Autodesk Inventor part; units mm, degrees
(part 2 of 5)
sketch "スケッチ2" plane through (0, 0, 0) normal (0, 0, 1) x (1, 0, 0)
  arc A0 (152.8433, 93.1355) -> (152.2497, 92.5446) centre (153.1871, 92.1964) ccw
  arc A1 (144.7503, 92.5446) -> (152.2497, 92.5446) centre (148.5, 93.9374) ccw
  arc A2 (144.7503, 92.5446) -> (144.1567, 93.1355) centre (143.8129, 92.1964) ccw
  arc A3 (143.2473, 93.5091) -> (144.1567, 93.1355) centre (148.5, 105) ccw
  arc A4 (142.7704, 93.9677) -> (143.2473, 93.5091) centre (143.663, 94.4186) ccw
  arc A5 (141.9213, 97.4341) -> (142.7704, 93.9677) centre (149.832, 97.5348) ccw
  arc A6 (141.9213, 97.4341) -> (140.9341, 98.4213) centre (140.9213, 97.4213) ccw
  arc A7 (137.4677, 99.2704) -> (140.9341, 98.4213) centre (141.0348, 106.332) ccw
  arc A8 (137.0091, 99.7473) -> (137.4677, 99.2704) centre (137.9186, 100.163) ccw
  arc A9 (136.6355, 100.6567) -> (137.0091, 99.7473) centre (148.5, 105) ccw
  arc A10 (136.6355, 100.6567) -> (136.0446, 101.2503) centre (135.6964, 100.3129) ccw
  arc A11 (136.0446, 108.7497) -> (136.0446, 101.2503) centre (137.4374, 105) ccw
  arc A12 (136.0446, 108.7497) -> (136.6355, 109.3433) centre (135.6964, 109.6871) ccw
  arc A13 (137.0091, 110.2527) -> (136.6355, 109.3433) centre (148.5, 105) ccw
  arc A14 (137.4677, 110.7296) -> (137.0091, 110.2527) centre (137.9186, 109.837) ccw
  arc A15 (140.9341, 111.5787) -> (137.4677, 110.7296) centre (141.0348, 103.668) ccw
  arc A16 (140.9341, 111.5787) -> (141.9213, 112.5659) centre (140.9213, 112.5787) ccw
  arc A17 (142.7704, 116.0323) -> (141.9213, 112.5659) centre (149.832, 112.4652) ccw
  arc A18 (143.2473, 116.4909) -> (142.7704, 116.0323) centre (143.663, 115.5814) ccw
  arc A19 (144.1567, 116.8645) -> (143.2473, 116.4909) centre (148.5, 105) ccw
  arc A20 (144.1567, 116.8645) -> (144.7503, 117.4554) centre (143.8129, 117.8036) ccw
  arc A21 (152.2497, 117.4554) -> (144.7503, 117.4554) centre (148.5, 116.0626) ccw
  arc A22 (152.2497, 117.4554) -> (152.8433, 116.8645) centre (153.1871, 117.8036) ccw
  arc A23 (153.7527, 116.4909) -> (152.8433, 116.8645) centre (148.5, 105) ccw
  arc A24 (154.2296, 116.0323) -> (153.7527, 116.4909) centre (153.337, 115.5814) ccw
  arc A25 (155.0787, 112.5659) -> (154.2296, 116.0323) centre (147.168, 112.4652) ccw
  arc A26 (155.0787, 112.5659) -> (156.0659, 111.5787) centre (156.0787, 112.5787) ccw
  arc A27 (159.5323, 110.7296) -> (156.0659, 111.5787) centre (155.9652, 103.668) ccw
  arc A28 (159.9909, 110.2527) -> (159.5323, 110.7296) centre (159.0814, 109.837) ccw
  arc A29 (160.3645, 109.3433) -> (159.9909, 110.2527) centre (148.5, 105) ccw
  arc A30 (160.3645, 109.3433) -> (160.9554, 108.7497) centre (161.3036, 109.6871) ccw
  arc A31 (160.9554, 101.2503) -> (160.9554, 108.7497) centre (159.5626, 105) ccw
  arc A32 (160.9554, 101.2503) -> (160.3645, 100.6567) centre (161.3036, 100.3129) ccw
  arc A33 (159.9909, 99.7473) -> (160.3645, 100.6567) centre (148.5, 105) ccw
  arc A34 (159.5323, 99.2704) -> (159.9909, 99.7473) centre (159.0814, 100.163) ccw
  arc A35 (156.0659, 98.4213) -> (159.5323, 99.2704) centre (155.9652, 106.332) ccw
  arc A36 (156.0659, 98.4213) -> (155.0787, 97.4341) centre (156.0787, 97.4213) ccw
  arc A37 (154.2296, 93.9677) -> (155.0787, 97.4341) centre (147.168, 97.5348) ccw
  arc A38 (153.7527, 93.5091) -> (154.2296, 93.9677) centre (153.337, 94.4186) ccw
  arc A39 (152.8433, 93.1355) -> (153.7527, 93.5091) centre (148.5, 105) ccw
  circle A40 centre (148.5, 105) radius 3
  circle A41 centre (148.5, 116.0626) radius 1.25
  circle A42 centre (137.4374, 105) radius 1.25
  circle A43 centre (159.5626, 105) radius 1.25
  circle A44 centre (148.5, 93.9374) radius 1.25
  arc A45 (148.106, 135.7475) -> (147.9566, 136.3017) centre (140.7163, 134.0527) ccw projected
  arc A46 (148.894, 135.7475) -> (148.106, 135.7475) centre (148.5, 105) ccw projected
  arc A47 (149.0434, 136.3017) -> (148.894, 135.7475) centre (156.2837, 134.0527) ccw projected
  arc A48 (149.3046, 137.0392) -> (149.0434, 136.3017) centre (158.5049, 133.3653) ccw projected
  arc A49 (149.7251, 137.9773) -> (149.3046, 137.0392) centre (160.7701, 132.4624) ccw projected
  arc A50 (150.5131, 137.9385) -> (149.7251, 137.9773) centre (148.5, 105) ccw projected
  arc A51 (150.8397, 136.9638) -> (150.5131, 137.9385) centre (138.9807, 133.5328) ccw projected
  arc A52 (151.0273, 136.2043) -> (150.8397, 136.9638) centre (141.3236, 134.2093) ccw projected
  arc A53 (151.1217, 135.638) -> (151.0273, 136.2043) centre (143.6015, 134.6758) ccw projected
  arc A54 (151.9058, 135.5608) -> (151.1217, 135.638) centre (148.5, 105) ccw projected
  arc A55 (152.1089, 136.0978) -> (151.9058, 135.5608) centre (159.0939, 133.1499) ccw projected
  arc A56 (152.4411, 136.8061) -> (152.1089, 136.0978) centre (161.237, 132.248) ccw projected
  arc A57 (152.9516, 137.6984) -> (152.4411, 136.8061) centre (163.4028, 131.1274) ccw projected
  arc A58 (153.7319, 137.5826) -> (152.9516, 137.6984) centre (148.5, 105) ccw projected
  arc A59 (153.9614, 136.5805) -> (153.7319, 137.5826) centre (141.8233, 134.3285) ccw projected
  arc A60 (154.0737, 135.8063) -> (153.9614, 136.5805) centre (144.2211, 134.7721) ccw projected
  arc A61 (154.1121, 135.2335) -> (154.0737, 135.8063) centre (146.5338, 135.013) ccw projected
  arc A62 (154.8849, 135.0798) -> (154.1121, 135.2335) centre (148.5, 105) ccw projected
  arc A63 (155.1396, 135.5943) -> (154.8849, 135.0798) centre (161.802, 131.976) ccw projected
  arc A64 (155.5397, 136.2666) -> (155.1396, 135.5943) centre (163.8464, 130.8684) ccw projected
  arc A65 (156.1351, 137.1046) -> (155.5397, 136.2666) centre (165.892, 129.5409) ccw projected
  arc A66 (156.9004, 136.9129) -> (156.1351, 137.1046) centre (148.5, 105) ccw projected
  arc A67 (157.0305, 135.8932) -> (156.9004, 136.9129) centre (144.7301, 134.8417) ccw projected
  arc A68 (157.0664, 135.1116) -> (157.0305, 135.8932) centre (147.1599, 135.0481) ccw projected
  arc A69 (157.0485, 134.5379) -> (157.0664, 135.1116) centre (149.485, 135.0612) ccw projected
  arc A70 (157.8025, 134.3091) -> (157.0485, 134.5379) centre (148.5, 105) ccw projected
  arc A71 (158.1064, 134.7962) -> (157.8025, 134.3091) centre (164.3821, 130.5422) ccw projected
  arc A72 (158.5704, 135.426) -> (158.1064, 134.7962) centre (166.3081, 129.2396) ccw projected
  arc A73 (159.2452, 136.2016) -> (158.5704, 135.426) centre (168.2137, 127.718) ccw projected
  arc A74 (159.988, 135.9358) -> (159.2452, 136.2016) centre (148.5, 105) ccw projected
  arc A75 (160.0175, 134.9083) -> (159.988, 135.9358) centre (147.6733, 135.0675) ccw projected
  arc A76 (159.9766, 134.127) -> (160.0175, 134.9083) centre (150.1116, 135.0348) ccw projected
  arc A77 (159.9026, 133.5577) -> (159.9766, 134.127) centre (152.4268, 134.8199) ccw projected
  arc A78 (160.6305, 133.2562) -> (159.9026, 133.5577) centre (148.5, 105) ccw projected
  arc A79 (160.9807, 133.7111) -> (160.6305, 133.2562) centre (166.8092, 128.8625) ccw projected
  arc A80 (161.5042, 134.2924) -> (160.9807, 133.7111) centre (168.5982, 127.3774) ccw projected
  arc A81 (162.2517, 134.9982) -> (161.5042, 134.2924) centre (170.3455, 125.6763) ccw projected
  arc A82 (162.9649, 134.6609) -> (162.2517, 134.9982) centre (148.5, 105) ccw projected
  arc A83 (162.8936, 133.6353) -> (162.9649, 134.6609) centre (150.6244, 135.0037) ccw projected
  arc A84 (162.7763, 132.8618) -> (162.8936, 133.6353) centre (153.0478, 134.7322) ccw projected
  arc A85 (162.6468, 132.3026) -> (162.7763, 132.8618) centre (155.3308, 134.2914) ccw projected
  arc A86 (163.3417, 131.9311) -> (162.6468, 132.3026) centre (148.5, 105) ccw projected
  arc A87 (163.7348, 132.3495) -> (163.3417, 131.9311) centre (169.06, 126.953) ccw projected
  arc A88 (164.3128, 132.8768) -> (163.7348, 132.3495) centre (170.6948, 125.2996) ccw projected
  arc A89 (165.1258, 133.5058) -> (164.3128, 132.8768) centre (172.267, 123.4355) ccw projected
  arc A90 (165.8025, 133.1002) -> (165.1258, 133.5058) centre (148.5, 105) ccw projected
  arc A91 (165.631, 132.0866) -> (165.8025, 133.1002) centre (153.555, 134.651) ccw projected
  arc A92 (165.4385, 131.3283) -> (165.631, 132.0866) centre (155.9401, 134.1433) ccw projected
  arc A93 (165.2548, 130.7845) -> (165.4385, 131.3283) centre (158.1689, 133.4809) ccw projected
  arc A94 (165.91, 130.3467) -> (165.2548, 130.7845) centre (148.5, 105) ccw projected
  arc A95 (166.3421, 130.7246) -> (165.91, 130.3467) centre (171.1127, 124.8321) ccw projected
  arc A96 (166.969, 131.1926) -> (166.3421, 130.7246) centre (172.5776, 123.0264) ccw projected
  arc A97 (167.8398, 131.7389) -> (166.969, 131.1926) centre (173.9595, 121.0172) ccw projected
  arc A98 (168.4735, 131.269) -> (167.8398, 131.7389) centre (148.5, 105) ccw projected
  arc A99 (168.2035, 130.2771) -> (168.4735, 131.269) centre (156.437, 134.0128) ccw projected
  arc A100 (167.9376, 129.5413) -> (168.2035, 130.2771) centre (158.7608, 133.2737) ccw projected
  arc A101 (167.7015, 129.018) -> (167.9376, 129.5413) centre (160.914, 132.396) ccw projected
  arc A102 (168.3105, 128.5182) -> (167.7015, 129.018) centre (148.5, 105) ccw projected
  arc A103 (168.7777, 128.8519) -> (168.3105, 128.5182) centre (172.9477, 122.5201) ccw projected
  arc A104 (169.4474, 129.2562) -> (168.7777, 128.8519) centre (174.2286, 120.5796) ccw projected
  arc A105 (170.3676, 129.7145) -> (169.4474, 129.2562) centre (175.4069, 118.4446) ccw projected
  arc A106 (170.9521, 129.1847) -> (170.3676, 129.7145) centre (148.5, 105) ccw projected
  arc A107 (170.5862, 128.2241) -> (170.9521, 129.1847) centre (159.2425, 133.0951) ccw projected
  arc A108 (170.2495, 127.5179) -> (170.5862, 128.2241) centre (161.4827, 132.1318) ccw projected
  arc A109 (169.9632, 127.0203) -> (170.2495, 127.5179) centre (163.5395, 131.0473) ccw projected
  arc A110 (170.5203, 126.4632) -> (169.9632, 127.0203) centre (148.5, 105) ccw projected
  arc A111 (171.0179, 126.7495) -> (170.5203, 126.4632) centre (174.5473, 120.0395) ccw projected
  arc A112 (171.7241, 127.0862) -> (171.0179, 126.7495) centre (175.6318, 117.9827) ccw projected
  arc A113 (172.6847, 127.4521) -> (171.7241, 127.0862) centre (176.5951, 115.7425) ccw projected
  arc A114 (173.2145, 126.8676) -> (172.6847, 127.4521) centre (148.5, 105) ccw projected
  arc A115 (172.7562, 125.9474) -> (173.2145, 126.8676) centre (161.9446, 131.9069) ccw projected
  arc A116 (172.3519, 125.2777) -> (172.7562, 125.9474) centre (164.0796, 130.7286) ccw projected
  arc A117 (172.0182, 124.8105) -> (172.3519, 125.2777) centre (166.0201, 129.4477) ccw projected
  arc A118 (172.518, 124.2015) -> (172.0182, 124.8105) centre (148.5, 105) ccw projected
  arc A119 (173.0413, 124.4376) -> (172.518, 124.2015) centre (175.896, 117.414) ccw projected
  arc A120 (173.7771, 124.7035) -> (173.0413, 124.4376) centre (176.7737, 115.2608) ccw projected
  arc A121 (174.769, 124.9735) -> (173.7771, 124.7035) centre (177.5128, 112.937) ccw projected
  arc A122 (175.2389, 124.3398) -> (174.769, 124.9735) centre (148.5, 105) ccw projected
  arc A123 (174.6926, 123.469) -> (175.2389, 124.3398) centre (164.5172, 130.4595) ccw projected
  arc A124 (174.2246, 122.8421) -> (174.6926, 123.469) centre (166.5264, 129.0776) ccw projected
  arc A125 (173.8467, 122.41) -> (174.2246, 122.8421) centre (168.3321, 127.6127) ccw projected
  arc A126 (174.2845, 121.7548) -> (173.8467, 122.41) centre (148.5, 105) ccw projected
  arc A127 (174.8283, 121.9385) -> (174.2845, 121.7548) centre (176.9809, 114.6689) ccw projected
  arc A128 (175.5866, 122.131) -> (174.8283, 121.9385) centre (177.6433, 112.4401) ccw projected
  arc A129 (176.6002, 122.3025) -> (175.5866, 122.131) centre (178.151, 110.055) ccw projected
  arc A130 (177.0058, 121.6258) -> (176.6002, 122.3025) centre (148.5, 105) ccw projected
  arc A131 (176.3768, 120.8128) -> (177.0058, 121.6258) centre (166.9355, 128.767) ccw projected
  arc A132 (175.8495, 120.2348) -> (176.3768, 120.8128) centre (168.7996, 127.1948) ccw projected
  arc A133 (175.4311, 119.8417) -> (175.8495, 120.2348) centre (170.453, 125.56) ccw projected
  arc A134 (175.8026, 119.1468) -> (175.4311, 119.8417) centre (148.5, 105) ccw projected
  arc A135 (176.3618, 119.2763) -> (175.8026, 119.1468) centre (177.7914, 111.8308) ccw projected
  arc A136 (177.1353, 119.3936) -> (176.3618, 119.2763) centre (178.2322, 109.5478) ccw projected
  arc A137 (178.1609, 119.4649) -> (177.1353, 119.3936) centre (178.5037, 107.1244) ccw projected
  arc A138 (178.4982, 118.7517) -> (178.1609, 119.4649) centre (148.5, 105) ccw projected
  arc A139 (177.7924, 118.0042) -> (178.4982, 118.7517) centre (169.1763, 126.8455) ccw projected
  arc A140 (177.2111, 117.4807) -> (177.7924, 118.0042) centre (170.8774, 125.0982) ccw projected
  arc A141 (176.7562, 117.1305) -> (177.2111, 117.4807) centre (172.3625, 123.3092) ccw projected
  arc A142 (177.0577, 116.4026) -> (176.7562, 117.1305) centre (148.5, 105) ccw projected
  arc A143 (177.627, 116.4766) -> (177.0577, 116.4026) centre (178.3199, 108.9268) ccw projected
  arc A144 (178.4083, 116.5175) -> (177.627, 116.4766) centre (178.5348, 106.6116) ccw projected
  arc A145 (179.4358, 116.488) -> (178.4083, 116.5175) centre (178.5675, 104.1733) ccw projected
  arc A146 (179.7016, 115.7452) -> (179.4358, 116.488) centre (148.5, 105) ccw projected
  arc A147 (178.926, 115.0704) -> (179.7016, 115.7452) centre (171.218, 124.7137) ccw projected
  arc A148 (178.2962, 114.6064) -> (178.926, 115.0704) centre (172.7396, 122.8081) ccw projected
  arc A149 (177.8091, 114.3025) -> (178.2962, 114.6064) centre (174.0422, 120.8821) ccw projected
  arc A150 (178.0379, 113.5485) -> (177.8091, 114.3025) centre (148.5, 105) ccw projected
  arc A151 (178.6116, 113.5664) -> (178.0379, 113.5485) centre (178.5612, 105.985) ccw projected
  arc A152 (179.3932, 113.5305) -> (178.6116, 113.5664) centre (178.5481, 103.6599) ccw projected
  arc A153 (180.4129, 113.4004) -> (179.3932, 113.5305) centre (178.3417, 101.2301) ccw projected
  arc A154 (180.6046, 112.6351) -> (180.4129, 113.4004) centre (148.5, 105) ccw projected
  arc A155 (179.7666, 112.0397) -> (180.6046, 112.6351) centre (173.0409, 122.392) ccw projected
  arc A156 (179.0943, 111.6396) -> (179.7666, 112.0397) centre (174.3684, 120.3464) ccw projected
  arc A157 (178.5798, 111.3849) -> (179.0943, 111.6396) centre (175.476, 118.302) ccw projected
  arc A158 (178.7335, 110.6121) -> (178.5798, 111.3849) centre (148.5, 105) ccw projected
  arc A159 (179.3063, 110.5737) -> (178.7335, 110.6121) centre (178.513, 103.0338) ccw projected
  arc A160 (180.0805, 110.4614) -> (179.3063, 110.5737) centre (178.2721, 100.7211) ccw projected
  arc A161 (181.0826, 110.2319) -> (180.0805, 110.4614) centre (177.8285, 98.3233) ccw projected
  arc A162 (181.1984, 109.4516) -> (181.0826, 110.2319) centre (148.5, 105) ccw projected
  arc A163 (180.3061, 108.9411) -> (181.1984, 109.4516) centre (174.6274, 119.9028) ccw projected
  arc A164 (179.5978, 108.6089) -> (180.3061, 108.9411) centre (175.748, 117.737) ccw projected
  arc A165 (179.0608, 108.4058) -> (179.5978, 108.6089) centre (176.6499, 115.5939) ccw projected
  arc A166 (179.138, 107.6217) -> (179.0608, 108.4058) centre (148.5, 105) ccw projected
  arc A167 (179.7043, 107.5273) -> (179.138, 107.6217) centre (178.1758, 100.1015) ccw projected
  arc A168 (180.4638, 107.3397) -> (179.7043, 107.5273) centre (177.7093, 97.8236) ccw projected
  arc A169 (181.4385, 107.0131) -> (180.4638, 107.3397) centre (177.0328, 95.4807) ccw projected
  arc A170 (181.4773, 106.2251) -> (181.4385, 107.0131) centre (148.5, 105) ccw projected
  arc A171 (180.5392, 105.8046) -> (181.4773, 106.2251) centre (175.9624, 117.2701) ccw projected
  arc A172 (179.8017, 105.5434) -> (180.5392, 105.8046) centre (176.8653, 115.0049) ccw projected
  arc A173 (179.2475, 105.394) -> (179.8017, 105.5434) centre (177.5527, 112.7837) ccw projected
  arc A174 (179.2475, 104.606) -> (179.2475, 105.394) centre (148.5, 105) ccw projected
  arc A175 (179.8017, 104.4566) -> (179.2475, 104.606) centre (177.5527, 97.2163) ccw projected
  arc A176 (180.5392, 104.1954) -> (179.8017, 104.4566) centre (176.8653, 94.9951) ccw projected
  arc A177 (181.4773, 103.7749) -> (180.5392, 104.1954) centre (175.9624, 92.7299) ccw projected
  arc A178 (181.4385, 102.9869) -> (181.4773, 103.7749) centre (148.5, 105) ccw projected
  arc A179 (180.4638, 102.6603) -> (181.4385, 102.9869) centre (177.0328, 114.5193) ccw projected
  arc A180 (179.7043, 102.4727) -> (180.4638, 102.6603) centre (177.7093, 112.1764) ccw projected
  arc A181 (179.138, 102.3783) -> (179.7043, 102.4727) centre (178.1758, 109.8985) ccw projected
  arc A182 (179.0608, 101.5942) -> (179.138, 102.3783) centre (148.5, 105) ccw projected
  arc A183 (179.5978, 101.3911) -> (179.0608, 101.5942) centre (176.6499, 94.4061) ccw projected
  arc A184 (180.3061, 101.0589) -> (179.5978, 101.3911) centre (175.748, 92.263) ccw projected
  arc A185 (181.1984, 100.5484) -> (180.3061, 101.0589) centre (174.6274, 90.0972) ccw projected
  arc A186 (181.0826, 99.7681) -> (181.1984, 100.5484) centre (148.5, 105) ccw projected
  arc A187 (180.0805, 99.5386) -> (181.0826, 99.7681) centre (177.8285, 111.6767) ccw projected
  arc A188 (179.3063, 99.4263) -> (180.0805, 99.5386) centre (178.2721, 109.2789) ccw projected
  arc A189 (178.7335, 99.3879) -> (179.3063, 99.4263) centre (178.513, 106.9662) ccw projected
  arc A190 (178.5798, 98.6151) -> (178.7335, 99.3879) centre (148.5, 105) ccw projected
  arc A191 (179.0943, 98.3604) -> (178.5798, 98.6151) centre (175.476, 91.698) ccw projected
  arc A192 (179.7666, 97.9603) -> (179.0943, 98.3604) centre (174.3684, 89.6536) ccw projected
  arc A193 (180.6046, 97.3649) -> (179.7666, 97.9603) centre (173.0409, 87.608) ccw projected
  arc A194 (180.4129, 96.5996) -> (180.6046, 97.3649) centre (148.5, 105) ccw projected
  arc A195 (179.3932, 96.4695) -> (180.4129, 96.5996) centre (178.3417, 108.7699) ccw projected
  arc A196 (178.6116, 96.4336) -> (179.3932, 96.4695) centre (178.5481, 106.3401) ccw projected
  arc A197 (178.0379, 96.4515) -> (178.6116, 96.4336) centre (178.5612, 104.015) ccw projected
  arc A198 (177.8091, 95.6975) -> (178.0379, 96.4515) centre (148.5, 105) ccw projected
  arc A199 (178.2962, 95.3936) -> (177.8091, 95.6975) centre (174.0422, 89.1179) ccw projected
  arc A200 (178.926, 94.9296) -> (178.2962, 95.3936) centre (172.7396, 87.1919) ccw projected
  arc A201 (179.7016, 94.2548) -> (178.926, 94.9296) centre (171.218, 85.2863) ccw projected
  arc A202 (179.4358, 93.512) -> (179.7016, 94.2548) centre (148.5, 105) ccw projected
  arc A203 (178.4083, 93.4825) -> (179.4358, 93.512) centre (178.5675, 105.8267) ccw projected
  arc A204 (177.627, 93.5234) -> (178.4083, 93.4825) centre (178.5348, 103.3884) ccw projected
  arc A205 (177.0577, 93.5974) -> (177.627, 93.5234) centre (178.3199, 101.0732) ccw projected
  arc A206 (176.7562, 92.8695) -> (177.0577, 93.5974) centre (148.5, 105) ccw projected
  arc A207 (177.2111, 92.5193) -> (176.7562, 92.8695) centre (172.3625, 86.6908) ccw projected
  arc A208 (177.7924, 91.9958) -> (177.2111, 92.5193) centre (170.8774, 84.9018) ccw projected
  arc A209 (178.4982, 91.2483) -> (177.7924, 91.9958) centre (169.1763, 83.1545) ccw projected
  arc A210 (178.1609, 90.5351) -> (178.4982, 91.2483) centre (148.5, 105) ccw projected
  arc A211 (177.1353, 90.6064) -> (178.1609, 90.5351) centre (178.5037, 102.8756) ccw projected
  arc A212 (176.3618, 90.7237) -> (177.1353, 90.6064) centre (178.2322, 100.4522) ccw projected
  arc A213 (175.8026, 90.8532) -> (176.3618, 90.7237) centre (177.7914, 98.1692) ccw projected
  arc A214 (175.4311, 90.1583) -> (175.8026, 90.8532) centre (148.5, 105) ccw projected
  arc A215 (175.8495, 89.7652) -> (175.4311, 90.1583) centre (170.453, 84.44) ccw projected
  arc A216 (176.3768, 89.1872) -> (175.8495, 89.7652) centre (168.7996, 82.8052) ccw projected
  arc A217 (177.0058, 88.3742) -> (176.3768, 89.1872) centre (166.9355, 81.233) ccw projected
  arc A218 (176.6002, 87.6975) -> (177.0058, 88.3742) centre (148.5, 105) ccw projected
  arc A219 (175.5866, 87.869) -> (176.6002, 87.6975) centre (178.151, 99.945) ccw projected
  arc A220 (174.8283, 88.0615) -> (175.5866, 87.869) centre (177.6433, 97.5599) ccw projected
  arc A221 (174.2845, 88.2452) -> (174.8283, 88.0615) centre (176.9809, 95.3311) ccw projected
  arc A222 (173.8467, 87.59) -> (174.2845, 88.2452) centre (148.5, 105) ccw projected
  arc A223 (174.2246, 87.1579) -> (173.8467, 87.59) centre (168.3321, 82.3873) ccw projected
  arc A224 (174.6926, 86.531) -> (174.2246, 87.1579) centre (166.5264, 80.9224) ccw projected
  arc A225 (175.2389, 85.6602) -> (174.6926, 86.531) centre (164.5172, 79.5405) ccw projected
  arc A226 (174.769, 85.0265) -> (175.2389, 85.6602) centre (148.5, 105) ccw projected
  arc A227 (173.7771, 85.2965) -> (174.769, 85.0265) centre (177.5128, 97.063) ccw projected
  arc A228 (173.0413, 85.5624) -> (173.7771, 85.2965) centre (176.7737, 94.7392) ccw projected
  arc A229 (172.518, 85.7985) -> (173.0413, 85.5624) centre (175.896, 92.586) ccw projected
  arc A230 (172.0182, 85.1895) -> (172.518, 85.7985) centre (148.5, 105) ccw projected
  arc A231 (172.3519, 84.7223) -> (172.0182, 85.1895) centre (166.0201, 80.5523) ccw projected
  arc A232 (172.7562, 84.0526) -> (172.3519, 84.7223) centre (164.0796, 79.2714) ccw projected
  arc A233 (173.2145, 83.1324) -> (172.7562, 84.0526) centre (161.9446, 78.0931) ccw projected
  arc A234 (172.6847, 82.5479) -> (173.2145, 83.1324) centre (148.5, 105) ccw projected
  arc A235 (171.7241, 82.9138) -> (172.6847, 82.5479) centre (176.5951, 94.2575) ccw projected
  arc A236 (171.0179, 83.2505) -> (171.7241, 82.9138) centre (175.6318, 92.0173) ccw projected
  arc A237 (170.5203, 83.5368) -> (171.0179, 83.2505) centre (174.5473, 89.9605) ccw projected
  arc A238 (169.9632, 82.9797) -> (170.5203, 83.5368) centre (148.5, 105) ccw projected
  arc A239 (170.2495, 82.4821) -> (169.9632, 82.9797) centre (163.5395, 78.9527) ccw projected
  arc A240 (170.5862, 81.7759) -> (170.2495, 82.4821) centre (161.4827, 77.8682) ccw projected
  arc A241 (170.9521, 80.8153) -> (170.5862, 81.7759) centre (159.2425, 76.9049) ccw projected
  arc A242 (170.3676, 80.2855) -> (170.9521, 80.8153) centre (148.5, 105) ccw projected
  arc A243 (169.4474, 80.7438) -> (170.3676, 80.2855) centre (175.4069, 91.5554) ccw projected
  arc A244 (168.7777, 81.1481) -> (169.4474, 80.7438) centre (174.2286, 89.4204) ccw projected
  arc A245 (168.3105, 81.4818) -> (168.7777, 81.1481) centre (172.9477, 87.4799) ccw projected
  arc A246 (167.7015, 80.982) -> (168.3105, 81.4818) centre (148.5, 105) ccw projected
  arc A247 (167.9376, 80.4587) -> (167.7015, 80.982) centre (160.914, 77.604) ccw projected
  arc A248 (168.2035, 79.7229) -> (167.9376, 80.4587) centre (158.7608, 76.7263) ccw projected
  arc A249 (168.4735, 78.731) -> (168.2035, 79.7229) centre (156.437, 75.9872) ccw projected
  arc A250 (167.8398, 78.2611) -> (168.4735, 78.731) centre (148.5, 105) ccw projected
  arc A251 (166.969, 78.8074) -> (167.8398, 78.2611) centre (173.9595, 88.9828) ccw projected
  arc A252 (166.3421, 79.2754) -> (166.969, 78.8074) centre (172.5776, 86.9736) ccw projected
  arc A253 (165.91, 79.6533) -> (166.3421, 79.2754) centre (171.1127, 85.1679) ccw projected
  arc A254 (165.2548, 79.2155) -> (165.91, 79.6533) centre (148.5, 105) ccw projected
  arc A255 (165.4385, 78.6717) -> (165.2548, 79.2155) centre (158.1689, 76.5191) ccw projected
  arc A256 (165.631, 77.9134) -> (165.4385, 78.6717) centre (155.9401, 75.8567) ccw projected
  arc A257 (165.8025, 76.8998) -> (165.631, 77.9134) centre (153.555, 75.349) ccw projected
  arc A258 (165.1258, 76.4942) -> (165.8025, 76.8998) centre (148.5, 105) ccw projected
  arc A259 (164.3128, 77.1232) -> (165.1258, 76.4942) centre (172.267, 86.5645) ccw projected
  arc A260 (163.7348, 77.6505) -> (164.3128, 77.1232) centre (170.6948, 84.7004) ccw projected
  arc A261 (163.3417, 78.0689) -> (163.7348, 77.6505) centre (169.06, 83.047) ccw projected
  arc A262 (162.6468, 77.6974) -> (163.3417, 78.0689) centre (148.5, 105) ccw projected
  arc A263 (162.7763, 77.1382) -> (162.6468, 77.6974) centre (155.3308, 75.7086) ccw projected
  arc A264 (162.8936, 76.3647) -> (162.7763, 77.1382) centre (153.0478, 75.2678) ccw projected
  arc A265 (162.9649, 75.3391) -> (162.8936, 76.3647) centre (150.6244, 74.9963) ccw projected
  arc A266 (162.2517, 75.0018) -> (162.9649, 75.3391) centre (148.5, 105) ccw projected
  arc A267 (161.5042, 75.7076) -> (162.2517, 75.0018) centre (170.3455, 84.3237) ccw projected
  arc A268 (160.9807, 76.2889) -> (161.5042, 75.7076) centre (168.5982, 82.6226) ccw projected
  arc A269 (160.6305, 76.7438) -> (160.9807, 76.2889) centre (166.8092, 81.1375) ccw projected
  arc A270 (159.9026, 76.4423) -> (160.6305, 76.7438) centre (148.5, 105) ccw projected
  arc A271 (159.9766, 75.873) -> (159.9026, 76.4423) centre (152.4268, 75.1801) ccw projected
  arc A272 (160.0175, 75.0917) -> (159.9766, 75.873) centre (150.1116, 74.9652) ccw projected
  arc A273 (159.988, 74.0642) -> (160.0175, 75.0917) centre (147.6733, 74.9325) ccw projected
  arc A274 (159.2452, 73.7984) -> (159.988, 74.0642) centre (148.5, 105) ccw projected
  arc A275 (158.5704, 74.574) -> (159.2452, 73.7984) centre (168.2137, 82.282) ccw projected
  arc A276 (158.1064, 75.2038) -> (158.5704, 74.574) centre (166.3081, 80.7604) ccw projected
  arc A277 (157.8025, 75.6909) -> (158.1064, 75.2038) centre (164.3821, 79.4578) ccw projected
  arc A278 (157.0485, 75.4621) -> (157.8025, 75.6909) centre (148.5, 105) ccw projected
  arc A279 (157.0664, 74.8884) -> (157.0485, 75.4621) centre (149.485, 74.9388) ccw projected
  arc A280 (157.0305, 74.1068) -> (157.0664, 74.8884) centre (147.1599, 74.9519) ccw projected
  arc A281 (156.9004, 73.0871) -> (157.0305, 74.1068) centre (144.7301, 75.1583) ccw projected
  arc A282 (156.1351, 72.8954) -> (156.9004, 73.0871) centre (148.5, 105) ccw projected
  arc A283 (155.5397, 73.7334) -> (156.1351, 72.8954) centre (165.892, 80.4591) ccw projected
  arc A284 (155.1396, 74.4057) -> (155.5397, 73.7334) centre (163.8464, 79.1316) ccw projected
  arc A285 (154.8849, 74.9202) -> (155.1396, 74.4057) centre (161.802, 78.024) ccw projected
  arc A286 (154.1121, 74.7665) -> (154.8849, 74.9202) centre (148.5, 105) ccw projected
  arc A287 (154.0737, 74.1937) -> (154.1121, 74.7665) centre (146.5338, 74.987) ccw projected
  arc A288 (153.9614, 73.4195) -> (154.0737, 74.1937) centre (144.2211, 75.2279) ccw projected
  arc A289 (153.7319, 72.4174) -> (153.9614, 73.4195) centre (141.8233, 75.6715) ccw projected
  arc A290 (152.9516, 72.3016) -> (153.7319, 72.4174) centre (148.5, 105) ccw projected
  arc A291 (152.4411, 73.1939) -> (152.9516, 72.3016) centre (163.4028, 78.8726) ccw projected
  arc A292 (152.1089, 73.9022) -> (152.4411, 73.1939) centre (161.237, 77.752) ccw projected
  arc A293 (151.9058, 74.4392) -> (152.1089, 73.9022) centre (159.0939, 76.8501) ccw projected
  arc A294 (151.1217, 74.362) -> (151.9058, 74.4392) centre (148.5, 105) ccw projected
  arc A295 (151.0273, 73.7957) -> (151.1217, 74.362) centre (143.6015, 75.3242) ccw projected
  arc A296 (150.8397, 73.0362) -> (151.0273, 73.7957) centre (141.3236, 75.7907) ccw projected
  arc A297 (150.5131, 72.0615) -> (150.8397, 73.0362) centre (138.9807, 76.4672) ccw projected
  arc A298 (149.7251, 72.0227) -> (150.5131, 72.0615) centre (148.5, 105) ccw projected
  arc A299 (149.3046, 72.9608) -> (149.7251, 72.0227) centre (160.7701, 77.5376) ccw projected
  arc A300 (149.0434, 73.6983) -> (149.3046, 72.9608) centre (158.5049, 76.6347) ccw projected
  arc A301 (148.894, 74.2525) -> (149.0434, 73.6983) centre (156.2837, 75.9473) ccw projected
  arc A302 (148.106, 74.2525) -> (148.894, 74.2525) centre (148.5, 105) ccw projected
  arc A303 (147.9566, 73.6983) -> (148.106, 74.2525) centre (140.7163, 75.9473) ccw projected
  arc A304 (147.6954, 72.9608) -> (147.9566, 73.6983) centre (138.4951, 76.6347) ccw projected
  arc A305 (147.2749, 72.0227) -> (147.6954, 72.9608) centre (136.2299, 77.5376) ccw projected
  arc A306 (146.4869, 72.0615) -> (147.2749, 72.0227) centre (148.5, 105) ccw projected
  arc A307 (146.1603, 73.0362) -> (146.4869, 72.0615) centre (158.0193, 76.4672) ccw projected
  arc A308 (145.9727, 73.7957) -> (146.1603, 73.0362) centre (155.6764, 75.7907) ccw projected
  arc A309 (145.8783, 74.362) -> (145.9727, 73.7957) centre (153.3985, 75.3242) ccw projected
  arc A310 (145.0942, 74.4392) -> (145.8783, 74.362) centre (148.5, 105) ccw projected
  arc A311 (144.8911, 73.9022) -> (145.0942, 74.4392) centre (137.9061, 76.8501) ccw projected
  arc A312 (144.5589, 73.1939) -> (144.8911, 73.9022) centre (135.763, 77.752) ccw projected
  arc A313 (144.0484, 72.3016) -> (144.5589, 73.1939) centre (133.5972, 78.8726) ccw projected
  arc A314 (143.2681, 72.4174) -> (144.0484, 72.3016) centre (148.5, 105) ccw projected
  arc A315 (143.0386, 73.4195) -> (143.2681, 72.4174) centre (155.1767, 75.6715) ccw projected
  arc A316 (142.9263, 74.1937) -> (143.0386, 73.4195) centre (152.7789, 75.2279) ccw projected
  arc A317 (142.8879, 74.7665) -> (142.9263, 74.1937) centre (150.4662, 74.987) ccw projected
  arc A318 (142.1151, 74.9202) -> (142.8879, 74.7665) centre (148.5, 105) ccw projected
  arc A319 (141.8604, 74.4057) -> (142.1151, 74.9202) centre (135.198, 78.024) ccw projected
  arc A320 (141.4603, 73.7334) -> (141.8604, 74.4057) centre (133.1536, 79.1316) ccw projected
  arc A321 (140.8649, 72.8954) -> (141.4603, 73.7334) centre (131.108, 80.4591) ccw projected
  arc A322 (140.0996, 73.0871) -> (140.8649, 72.8954) centre (148.5, 105) ccw projected
  arc A323 (139.9695, 74.1068) -> (140.0996, 73.0871) centre (152.2699, 75.1583) ccw projected
  arc A324 (139.9336, 74.8884) -> (139.9695, 74.1068) centre (149.8401, 74.9519) ccw projected
  arc A325 (139.9515, 75.4621) -> (139.9336, 74.8884) centre (147.515, 74.9388) ccw projected
  arc A326 (139.1975, 75.6909) -> (139.9515, 75.4621) centre (148.5, 105) ccw projected
  arc A327 (138.8936, 75.2038) -> (139.1975, 75.6909) centre (132.6179, 79.4578) ccw projected
  arc A328 (138.4296, 74.574) -> (138.8936, 75.2038) centre (130.6919, 80.7604) ccw projected
  arc A329 (137.7548, 73.7984) -> (138.4296, 74.574) centre (128.7863, 82.282) ccw projected
  arc A330 (137.012, 74.0642) -> (137.7548, 73.7984) centre (148.5, 105) ccw projected
  arc A331 (136.9825, 75.0917) -> (137.012, 74.0642) centre (149.3267, 74.9325) ccw projected
  arc A332 (137.0234, 75.873) -> (136.9825, 75.0917) centre (146.8884, 74.9652) ccw projected
  arc A333 (137.0974, 76.4423) -> (137.0234, 75.873) centre (144.5732, 75.1801) ccw projected
  arc A334 (136.3695, 76.7438) -> (137.0974, 76.4423) centre (148.5, 105) ccw projected
  arc A335 (136.0193, 76.2889) -> (136.3695, 76.7438) centre (130.1908, 81.1375) ccw projected
  arc A336 (135.4958, 75.7076) -> (136.0193, 76.2889) centre (128.4018, 82.6226) ccw projected
  arc A337 (134.7483, 75.0018) -> (135.4958, 75.7076) centre (126.6545, 84.3237) ccw projected
  arc A338 (134.0351, 75.3391) -> (134.7483, 75.0018) centre (148.5, 105) ccw projected
  arc A339 (134.1064, 76.3647) -> (134.0351, 75.3391) centre (146.3756, 74.9963) ccw projected
  arc A340 (134.2237, 77.1382) -> (134.1064, 76.3647) centre (143.9522, 75.2678) ccw projected
  arc A341 (134.3532, 77.6974) -> (134.2237, 77.1382) centre (141.6692, 75.7086) ccw projected
  arc A342 (133.6583, 78.0689) -> (134.3532, 77.6974) centre (148.5, 105) ccw projected
  arc A343 (133.2652, 77.6505) -> (133.6583, 78.0689) centre (127.94, 83.047) ccw projected
  arc A344 (132.6872, 77.1232) -> (133.2652, 77.6505) centre (126.3052, 84.7004) ccw projected
  arc A345 (131.8742, 76.4942) -> (132.6872, 77.1232) centre (124.733, 86.5645) ccw projected
  arc A346 (131.1975, 76.8998) -> (131.8742, 76.4942) centre (148.5, 105) ccw projected
  arc A347 (131.369, 77.9134) -> (131.1975, 76.8998) centre (143.445, 75.349) ccw projected
  arc A348 (131.5615, 78.6717) -> (131.369, 77.9134) centre (141.0599, 75.8567) ccw projected
  arc A349 (131.7452, 79.2155) -> (131.5615, 78.6717) centre (138.8311, 76.5191) ccw projected
  arc A350 (131.09, 79.6533) -> (131.7452, 79.2155) centre (148.5, 105) ccw projected
  arc A351 (130.6579, 79.2754) -> (131.09, 79.6533) centre (125.8873, 85.1679) ccw projected
  arc A352 (130.031, 78.8074) -> (130.6579, 79.2754) centre (124.4224, 86.9736) ccw projected
  arc A353 (129.1602, 78.2611) -> (130.031, 78.8074) centre (123.0405, 88.9828) ccw projected
  arc A354 (128.5265, 78.731) -> (129.1602, 78.2611) centre (148.5, 105) ccw projected
  arc A355 (128.7965, 79.7229) -> (128.5265, 78.731) centre (140.563, 75.9872) ccw projected
  arc A356 (129.0624, 80.4587) -> (128.7965, 79.7229) centre (138.2392, 76.7263) ccw projected
  arc A357 (129.2985, 80.982) -> (129.0624, 80.4587) centre (136.086, 77.604) ccw projected
  arc A358 (128.6895, 81.4818) -> (129.2985, 80.982) centre (148.5, 105) ccw projected
  arc A359 (128.2223, 81.1481) -> (128.6895, 81.4818) centre (124.0523, 87.4799) ccw projected
  arc A360 (127.5526, 80.7438) -> (128.2223, 81.1481) centre (122.7714, 89.4204) ccw projected
  arc A361 (126.6324, 80.2855) -> (127.5526, 80.7438) centre (121.5931, 91.5554) ccw projected
  arc A362 (126.0479, 80.8153) -> (126.6324, 80.2855) centre (148.5, 105) ccw projected
  arc A363 (126.4138, 81.7759) -> (126.0479, 80.8153) centre (137.7575, 76.9049) ccw projected
  arc A364 (126.7505, 82.4821) -> (126.4138, 81.7759) centre (135.5173, 77.8682) ccw projected
  arc A365 (127.0368, 82.9797) -> (126.7505, 82.4821) centre (133.4605, 78.9527) ccw projected
  arc A366 (126.4797, 83.5368) -> (127.0368, 82.9797) centre (148.5, 105) ccw projected
  arc A367 (125.9821, 83.2505) -> (126.4797, 83.5368) centre (122.4527, 89.9605) ccw projected
  arc A368 (125.2759, 82.9138) -> (125.9821, 83.2505) centre (121.3682, 92.0173) ccw projected
  arc A369 (124.3153, 82.5479) -> (125.2759, 82.9138) centre (120.4049, 94.2575) ccw projected
  arc A370 (123.7855, 83.1324) -> (124.3153, 82.5479) centre (148.5, 105) ccw projected
  arc A371 (124.2438, 84.0526) -> (123.7855, 83.1324) centre (135.0554, 78.0931) ccw projected
  arc A372 (124.6481, 84.7223) -> (124.2438, 84.0526) centre (132.9204, 79.2714) ccw projected
  arc A373 (124.9818, 85.1895) -> (124.6481, 84.7223) centre (130.9799, 80.5523) ccw projected
  arc A374 (124.482, 85.7985) -> (124.9818, 85.1895) centre (148.5, 105) ccw projected
  arc A375 (123.9587, 85.5624) -> (124.482, 85.7985) centre (121.104, 92.586) ccw projected
  arc A376 (123.2229, 85.2965) -> (123.9587, 85.5624) centre (120.2263, 94.7392) ccw projected
  arc A377 (122.231, 85.0265) -> (123.2229, 85.2965) centre (119.4872, 97.063) ccw projected
  arc A378 (121.7611, 85.6602) -> (122.231, 85.0265) centre (148.5, 105) ccw projected
  arc A379 (122.3074, 86.531) -> (121.7611, 85.6602) centre (132.4828, 79.5405) ccw projected
  arc A380 (122.7754, 87.1579) -> (122.3074, 86.531) centre (130.4736, 80.9224) ccw projected
  arc A381 (123.1533, 87.59) -> (122.7754, 87.1579) centre (128.6679, 82.3873) ccw projected
  arc A382 (122.7155, 88.2452) -> (123.1533, 87.59) centre (148.5, 105) ccw projected
  arc A383 (122.1717, 88.0615) -> (122.7155, 88.2452) centre (120.0191, 95.3311) ccw projected
  arc A384 (121.4134, 87.869) -> (122.1717, 88.0615) centre (119.3567, 97.5599) ccw projected
  arc A385 (120.3998, 87.6975) -> (121.4134, 87.869) centre (118.849, 99.945) ccw projected
  arc A386 (119.9942, 88.3742) -> (120.3998, 87.6975) centre (148.5, 105) ccw projected
  arc A387 (120.6232, 89.1872) -> (119.9942, 88.3742) centre (130.0645, 81.233) ccw projected
  arc A388 (121.1505, 89.7652) -> (120.6232, 89.1872) centre (128.2004, 82.8052) ccw projected
  arc A389 (121.5689, 90.1583) -> (121.1505, 89.7652) centre (126.547, 84.44) ccw projected
  arc A390 (121.1974, 90.8532) -> (121.5689, 90.1583) centre (148.5, 105) ccw projected
  arc A391 (120.6382, 90.7237) -> (121.1974, 90.8532) centre (119.2086, 98.1692) ccw projected
  arc A392 (119.8647, 90.6064) -> (120.6382, 90.7237) centre (118.7678, 100.4522) ccw projected
  arc A393 (118.8391, 90.5351) -> (119.8647, 90.6064) centre (118.4963, 102.8756) ccw projected
  arc A394 (118.5018, 91.2483) -> (118.8391, 90.5351) centre (148.5, 105) ccw projected
  arc A395 (119.2076, 91.9958) -> (118.5018, 91.2483) centre (127.8237, 83.1545) ccw projected
  arc A396 (119.7889, 92.5193) -> (119.2076, 91.9958) centre (126.1226, 84.9018) ccw projected
  arc A397 (120.2438, 92.8695) -> (119.7889, 92.5193) centre (124.6375, 86.6908) ccw projected
  arc A398 (119.9423, 93.5974) -> (120.2438, 92.8695) centre (148.5, 105) ccw projected
  arc A399 (119.373, 93.5234) -> (119.9423, 93.5974) centre (118.6801, 101.0732) ccw projected
  arc A400 (118.5917, 93.4825) -> (119.373, 93.5234) centre (118.4652, 103.3884) ccw projected
  arc A401 (117.5642, 93.512) -> (118.5917, 93.4825) centre (118.4325, 105.8267) ccw projected
  arc A402 (117.2984, 94.2548) -> (117.5642, 93.512) centre (148.5, 105) ccw projected
  arc A403 (118.074, 94.9296) -> (117.2984, 94.2548) centre (125.782, 85.2863) ccw projected
  arc A404 (118.7038, 95.3936) -> (118.074, 94.9296) centre (124.2604, 87.1919) ccw projected
  arc A405 (119.1909, 95.6975) -> (118.7038, 95.3936) centre (122.9578, 89.1179) ccw projected
  arc A406 (118.9621, 96.4515) -> (119.1909, 95.6975) centre (148.5, 105) ccw projected
  arc A407 (118.3884, 96.4336) -> (118.9621, 96.4515) centre (118.4388, 104.015) ccw projected
  arc A408 (117.6068, 96.4695) -> (118.3884, 96.4336) centre (118.4519, 106.3401) ccw projected
  arc A409 (116.5871, 96.5996) -> (117.6068, 96.4695) centre (118.6583, 108.7699) ccw projected
  arc A410 (116.3954, 97.3649) -> (116.5871, 96.5996) centre (148.5, 105) ccw projected
  arc A411 (117.2334, 97.9603) -> (116.3954, 97.3649) centre (123.9591, 87.608) ccw projected
  arc A412 (117.9057, 98.3604) -> (117.2334, 97.9603) centre (122.6316, 89.6536) ccw projected
  arc A413 (118.4202, 98.6151) -> (117.9057, 98.3604) centre (121.524, 91.698) ccw projected
  arc A414 (118.2665, 99.3879) -> (118.4202, 98.6151) centre (148.5, 105) ccw projected
  arc A415 (117.6937, 99.4263) -> (118.2665, 99.3879) centre (118.487, 106.9662) ccw projected
  arc A416 (116.9195, 99.5386) -> (117.6937, 99.4263) centre (118.7279, 109.2789) ccw projected
  arc A417 (115.9174, 99.7681) -> (116.9195, 99.5386) centre (119.1715, 111.6767) ccw projected
  arc A418 (115.8016, 100.5484) -> (115.9174, 99.7681) centre (148.5, 105) ccw projected
  arc A419 (116.6939, 101.0589) -> (115.8016, 100.5484) centre (122.3726, 90.0972) ccw projected
  arc A420 (117.4022, 101.3911) -> (116.6939, 101.0589) centre (121.252, 92.263) ccw projected
  arc A421 (117.9392, 101.5942) -> (117.4022, 101.3911) centre (120.3501, 94.4061) ccw projected
  arc A422 (117.862, 102.3783) -> (117.9392, 101.5942) centre (148.5, 105) ccw projected
  arc A423 (117.2957, 102.4727) -> (117.862, 102.3783) centre (118.8242, 109.8985) ccw projected
  arc A424 (116.5362, 102.6603) -> (117.2957, 102.4727) centre (119.2907, 112.1764) ccw projected
  arc A425 (115.5615, 102.9869) -> (116.5362, 102.6603) centre (119.9672, 114.5193) ccw projected
  arc A426 (115.5227, 103.7749) -> (115.5615, 102.9869) centre (148.5, 105) ccw projected
  arc A427 (116.4608, 104.1954) -> (115.5227, 103.7749) centre (121.0376, 92.7299) ccw projected
  arc A428 (117.1983, 104.4566) -> (116.4608, 104.1954) centre (120.1347, 94.9951) ccw projected
  arc A429 (117.7525, 104.606) -> (117.1983, 104.4566) centre (119.4473, 97.2163) ccw projected
  arc A430 (117.7525, 105.394) -> (117.7525, 104.606) centre (148.5, 105) ccw projected
  arc A431 (117.1983, 105.5434) -> (117.7525, 105.394) centre (119.4473, 112.7837) ccw projected
  arc A432 (116.4608, 105.8046) -> (117.1983, 105.5434) centre (120.1347, 115.0049) ccw projected
  arc A433 (115.5227, 106.2251) -> (116.4608, 105.8046) centre (121.0376, 117.2701) ccw projected
  arc A434 (115.5615, 107.0131) -> (115.5227, 106.2251) centre (148.5, 105) ccw projected
  arc A435 (116.5362, 107.3397) -> (115.5615, 107.0131) centre (119.9672, 95.4807) ccw projected
  arc A436 (117.2957, 107.5273) -> (116.5362, 107.3397) centre (119.2907, 97.8236) ccw projected
  arc A437 (117.862, 107.6217) -> (117.2957, 107.5273) centre (118.8242, 100.1015) ccw projected
  arc A438 (117.9392, 108.4058) -> (117.862, 107.6217) centre (148.5, 105) ccw projected
  arc A439 (117.4022, 108.6089) -> (117.9392, 108.4058) centre (120.3501, 115.5939) ccw projected
  arc A440 (116.6939, 108.9411) -> (117.4022, 108.6089) centre (121.252, 117.737) ccw projected
  arc A441 (115.8016, 109.4516) -> (116.6939, 108.9411) centre (122.3726, 119.9028) ccw projected
  arc A442 (115.9174, 110.2319) -> (115.8016, 109.4516) centre (148.5, 105) ccw projected
  arc A443 (116.9195, 110.4614) -> (115.9174, 110.2319) centre (119.1715, 98.3233) ccw projected
  arc A444 (117.6937, 110.5737) -> (116.9195, 110.4614) centre (118.7279, 100.7211) ccw projected
  arc A445 (118.2665, 110.6121) -> (117.6937, 110.5737) centre (118.487, 103.0338) ccw projected
  arc A446 (118.4202, 111.3849) -> (118.2665, 110.6121) centre (148.5, 105) ccw projected
  arc A447 (117.9057, 111.6396) -> (118.4202, 111.3849) centre (121.524, 118.302) ccw projected
  arc A448 (117.2334, 112.0397) -> (117.9057, 111.6396) centre (122.6316, 120.3464) ccw projected
  arc A449 (116.3954, 112.6351) -> (117.2334, 112.0397) centre (123.9591, 122.392) ccw projected
  arc A450 (116.5871, 113.4004) -> (116.3954, 112.6351) centre (148.5, 105) ccw projected
  arc A451 (117.6068, 113.5305) -> (116.5871, 113.4004) centre (118.6583, 101.2301) ccw projected
  arc A452 (118.3884, 113.5664) -> (117.6068, 113.5305) centre (118.4519, 103.6599) ccw projected
  arc A453 (118.9621, 113.5485) -> (118.3884, 113.5664) centre (118.4388, 105.985) ccw projected
  arc A454 (119.1909, 114.3025) -> (118.9621, 113.5485) centre (148.5, 105) ccw projected
  arc A455 (118.7038, 114.6064) -> (119.1909, 114.3025) centre (122.9578, 120.8821) ccw projected
  arc A456 (118.074, 115.0704) -> (118.7038, 114.6064) centre (124.2604, 122.8081) ccw projected
  arc A457 (117.2984, 115.7452) -> (118.074, 115.0704) centre (125.782, 124.7137) ccw projected
  arc A458 (117.5642, 116.488) -> (117.2984, 115.7452) centre (148.5, 105) ccw projected
  arc A459 (118.5917, 116.5175) -> (117.5642, 116.488) centre (118.4325, 104.1733) ccw projected
  arc A460 (119.373, 116.4766) -> (118.5917, 116.5175) centre (118.4652, 106.6116) ccw projected
  arc A461 (119.9423, 116.4026) -> (119.373, 116.4766) centre (118.6801, 108.9268) ccw projected
  arc A462 (120.2438, 117.1305) -> (119.9423, 116.4026) centre (148.5, 105) ccw projected
  arc A463 (119.7889, 117.4807) -> (120.2438, 117.1305) centre (124.6375, 123.3092) ccw projected
  arc A464 (119.2076, 118.0042) -> (119.7889, 117.4807) centre (126.1226, 125.0982) ccw projected
  arc A465 (118.5018, 118.7517) -> (119.2076, 118.0042) centre (127.8237, 126.8455) ccw projected
  arc A466 (118.8391, 119.4649) -> (118.5018, 118.7517) centre (148.5, 105) ccw projected
  arc A467 (119.8647, 119.3936) -> (118.8391, 119.4649) centre (118.4963, 107.1244) ccw projected
  arc A468 (120.6382, 119.2763) -> (119.8647, 119.3936) centre (118.7678, 109.5478) ccw projected
  arc A469 (121.1974, 119.1468) -> (120.6382, 119.2763) centre (119.2086, 111.8308) ccw projected
  arc A470 (121.5689, 119.8417) -> (121.1974, 119.1468) centre (148.5, 105) ccw projected
  arc A471 (121.1505, 120.2348) -> (121.5689, 119.8417) centre (126.547, 125.56) ccw projected
  arc A472 (120.6232, 120.8128) -> (121.1505, 120.2348) centre (128.2004, 127.1948) ccw projected
  arc A473 (119.9942, 121.6258) -> (120.6232, 120.8128) centre (130.0645, 128.767) ccw projected
  arc A474 (120.3998, 122.3025) -> (119.9942, 121.6258) centre (148.5, 105) ccw projected
  arc A475 (121.4134, 122.131) -> (120.3998, 122.3025) centre (118.849, 110.055) ccw projected
  arc A476 (122.1717, 121.9385) -> (121.4134, 122.131) centre (119.3567, 112.4401) ccw projected
  arc A477 (122.7155, 121.7548) -> (122.1717, 121.9385) centre (120.0191, 114.6689) ccw projected
  arc A478 (123.1533, 122.41) -> (122.7155, 121.7548) centre (148.5, 105) ccw projected
  arc A479 (122.7754, 122.8421) -> (123.1533, 122.41) centre (128.6679, 127.6127) ccw projected
  arc A480 (122.3074, 123.469) -> (122.7754, 122.8421) centre (130.4736, 129.0776) ccw projected
  arc A481 (121.7611, 124.3398) -> (122.3074, 123.469) centre (132.4828, 130.4595) ccw projected
  arc A482 (122.231, 124.9735) -> (121.7611, 124.3398) centre (148.5, 105) ccw projected
  arc A483 (123.2229, 124.7035) -> (122.231, 124.9735) centre (119.4872, 112.937) ccw projected
  arc A484 (123.9587, 124.4376) -> (123.2229, 124.7035) centre (120.2263, 115.2608) ccw projected
  arc A485 (124.482, 124.2015) -> (123.9587, 124.4376) centre (121.104, 117.414) ccw projected
  arc A486 (124.9818, 124.8105) -> (124.482, 124.2015) centre (148.5, 105) ccw projected
  arc A487 (124.6481, 125.2777) -> (124.9818, 124.8105) centre (130.9799, 129.4477) ccw projected
  arc A488 (124.2438, 125.9474) -> (124.6481, 125.2777) centre (132.9204, 130.7286) ccw projected
  arc A489 (123.7855, 126.8676) -> (124.2438, 125.9474) centre (135.0554, 131.9069) ccw projected
  arc A490 (124.3153, 127.4521) -> (123.7855, 126.8676) centre (148.5, 105) ccw projected
  arc A491 (125.2759, 127.0862) -> (124.3153, 127.4521) centre (120.4049, 115.7425) ccw projected
  arc A492 (125.9821, 126.7495) -> (125.2759, 127.0862) centre (121.3682, 117.9827) ccw projected
  arc A493 (126.4797, 126.4632) -> (125.9821, 126.7495) centre (122.4527, 120.0395) ccw projected
  arc A494 (127.0368, 127.0203) -> (126.4797, 126.4632) centre (148.5, 105) ccw projected
  arc A495 (126.7505, 127.5179) -> (127.0368, 127.0203) centre (133.4605, 131.0473) ccw projected
  arc A496 (126.4138, 128.2241) -> (126.7505, 127.5179) centre (135.5173, 132.1318) ccw projected
  arc A497 (126.0479, 129.1847) -> (126.4138, 128.2241) centre (137.7575, 133.0951) ccw projected
  arc A498 (126.6324, 129.7145) -> (126.0479, 129.1847) centre (148.5, 105) ccw projected
  arc A499 (127.5526, 129.2562) -> (126.6324, 129.7145) centre (121.5931, 118.4446) ccw projected
  arc A500 (128.2223, 128.8519) -> (127.5526, 129.2562) centre (122.7714, 120.5796) ccw projected
  arc A501 (128.6895, 128.5182) -> (128.2223, 128.8519) centre (124.0523, 122.5201) ccw projected
  arc A502 (129.2985, 129.018) -> (128.6895, 128.5182) centre (148.5, 105) ccw projected
  arc A503 (129.0624, 129.5413) -> (129.2985, 129.018) centre (136.086, 132.396) ccw projected
  arc A504 (128.7965, 130.2771) -> (129.0624, 129.5413) centre (138.2392, 133.2737) ccw projected
  arc A505 (128.5265, 131.269) -> (128.7965, 130.2771) centre (140.563, 134.0128) ccw projected
  arc A506 (129.1602, 131.7389) -> (128.5265, 131.269) centre (148.5, 105) ccw projected
  arc A507 (130.031, 131.1926) -> (129.1602, 131.7389) centre (123.0405, 121.0172) ccw projected
  arc A508 (130.6579, 130.7246) -> (130.031, 131.1926) centre (124.4224, 123.0264) ccw projected
  arc A509 (131.09, 130.3467) -> (130.6579, 130.7246) centre (125.8873, 124.8321) ccw projected
  arc A510 (131.7452, 130.7845) -> (131.09, 130.3467) centre (148.5, 105) ccw projected
  arc A511 (131.5615, 131.3283) -> (131.7452, 130.7845) centre (138.8311, 133.4809) ccw projected
  arc A512 (131.369, 132.0866) -> (131.5615, 131.3283) centre (141.0599, 134.1433) ccw projected
  arc A513 (131.1975, 133.1002) -> (131.369, 132.0866) centre (143.445, 134.651) ccw projected
  arc A514 (131.8742, 133.5058) -> (131.1975, 133.1002) centre (148.5, 105) ccw projected
  arc A515 (132.6872, 132.8768) -> (131.8742, 133.5058) centre (124.733, 123.4355) ccw projected
  arc A516 (133.2652, 132.3495) -> (132.6872, 132.8768) centre (126.3052, 125.2996) ccw projected
  arc A517 (133.6583, 131.9311) -> (133.2652, 132.3495) centre (127.94, 126.953) ccw projected
  arc A518 (134.3532, 132.3026) -> (133.6583, 131.9311) centre (148.5, 105) ccw projected
  arc A519 (134.2237, 132.8618) -> (134.3532, 132.3026) centre (141.6692, 134.2914) ccw projected
  arc A520 (134.1064, 133.6353) -> (134.2237, 132.8618) centre (143.9522, 134.7322) ccw projected
  arc A521 (134.0351, 134.6609) -> (134.1064, 133.6353) centre (146.3756, 135.0037) ccw projected
  arc A522 (134.7483, 134.9982) -> (134.0351, 134.6609) centre (148.5, 105) ccw projected
  arc A523 (135.4958, 134.2924) -> (134.7483, 134.9982) centre (126.6545, 125.6763) ccw projected
  arc A524 (136.0193, 133.7111) -> (135.4958, 134.2924) centre (128.4018, 127.3774) ccw projected
  arc A525 (136.3695, 133.2562) -> (136.0193, 133.7111) centre (130.1908, 128.8625) ccw projected
  arc A526 (137.0974, 133.5577) -> (136.3695, 133.2562) centre (148.5, 105) ccw projected
  arc A527 (137.0234, 134.127) -> (137.0974, 133.5577) centre (144.5732, 134.8199) ccw projected
  arc A528 (136.9825, 134.9083) -> (137.0234, 134.127) centre (146.8884, 135.0348) ccw projected
  arc A529 (137.012, 135.9358) -> (136.9825, 134.9083) centre (149.3267, 135.0675) ccw projected
  arc A530 (137.7548, 136.2016) -> (137.012, 135.9358) centre (148.5, 105) ccw projected
  arc A531 (138.4296, 135.426) -> (137.7548, 136.2016) centre (128.7863, 127.718) ccw projected
  arc A532 (138.8936, 134.7962) -> (138.4296, 135.426) centre (130.6919, 129.2396) ccw projected
  arc A533 (139.1975, 134.3091) -> (138.8936, 134.7962) centre (132.6179, 130.5422) ccw projected
  arc A534 (139.9515, 134.5379) -> (139.1975, 134.3091) centre (148.5, 105) ccw projected
  arc A535 (139.9336, 135.1116) -> (139.9515, 134.5379) centre (147.515, 135.0612) ccw projected
  arc A536 (139.9695, 135.8932) -> (139.9336, 135.1116) centre (149.8401, 135.0481) ccw projected
  arc A537 (140.0996, 136.9129) -> (139.9695, 135.8932) centre (152.2699, 134.8417) ccw projected
  arc A538 (140.8649, 137.1046) -> (140.0996, 136.9129) centre (148.5, 105) ccw projected
  arc A539 (141.4603, 136.2666) -> (140.8649, 137.1046) centre (131.108, 129.5409) ccw projected
  arc A540 (141.8604, 135.5943) -> (141.4603, 136.2666) centre (133.1536, 130.8684) ccw projected
  arc A541 (142.1151, 135.0798) -> (141.8604, 135.5943) centre (135.198, 131.976) ccw projected
  arc A542 (142.8879, 135.2335) -> (142.1151, 135.0798) centre (148.5, 105) ccw projected
  arc A543 (142.9263, 135.8063) -> (142.8879, 135.2335) centre (150.4662, 135.013) ccw projected
  arc A544 (143.0386, 136.5805) -> (142.9263, 135.8063) centre (152.7789, 134.7721) ccw projected
  arc A545 (143.2681, 137.5826) -> (143.0386, 136.5805) centre (155.1767, 134.3285) ccw projected
  arc A546 (144.0484, 137.6984) -> (143.2681, 137.5826) centre (148.5, 105) ccw projected
  arc A547 (144.5589, 136.8061) -> (144.0484, 137.6984) centre (133.5972, 131.1274) ccw projected
  arc A548 (144.8911, 136.0978) -> (144.5589, 136.8061) centre (135.763, 132.248) ccw projected
  arc A549 (145.0942, 135.5608) -> (144.8911, 136.0978) centre (137.9061, 133.1499) ccw projected
  arc A550 (145.8783, 135.638) -> (145.0942, 135.5608) centre (148.5, 105) ccw projected
  arc A551 (145.9727, 136.2043) -> (145.8783, 135.638) centre (153.3985, 134.6758) ccw projected
  arc A552 (146.1603, 136.9638) -> (145.9727, 136.2043) centre (155.6764, 134.2093) ccw projected
  arc A553 (146.4869, 137.9385) -> (146.1603, 136.9638) centre (158.0193, 133.5328) ccw projected
  arc A554 (147.2749, 137.9773) -> (146.4869, 137.9385) centre (148.5, 105) ccw projected
  arc A555 (147.6954, 137.0392) -> (147.2749, 137.9773) centre (136.2299, 132.4624) ccw projected
  arc A556 (147.9566, 136.3017) -> (147.6954, 137.0392) centre (138.4951, 133.3653) ccw projected
  point P0 (0, 0)
  point P1 (0, 0)
  constraints: 80 point on circle, 45 centre point, 258 other
extrude "押し出し2" cut sketch "スケッチ2" against normal blind 10 contours A40
extrude "押し出し3" cut sketch "スケッチ2" against normal blind 10 contours A41 | A42 | A43 | A44
extrude "押し出し4" cut sketch "スケッチ2" against normal blind 2.5 contours A0 A1 A2 A3 A4 A5 A6 A7 A8 A9 A10 A11 A12 A13 A14 A15 A16 A17 A18 A19 A20 A21 A22 A23 A24 A25 A26 A27 A28 A29 A30 A31 A32 A33 A34 A35 A36 A37 A38 A39